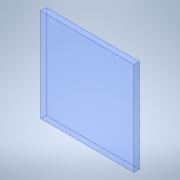
# Autodesk Inventor part: 20_cube_circular_polarizer
Saved by Autodesk Inventor 2022 (Build 260153000, 153)
## iProperties
Created: 2020-10-09
Part Number: 20_cube_circular_polarizer
Material: Generisch
Document SubType Name: Blech
Designer: UC2
Density: 1 g/cm^3
Sheet Metal Rule: Default
Appearance: Vorgabe
Author: UC2
Autodesk Inventor part; units mm, degrees
ref_plane "YZ Plane" through (0, 0, 0) normal (1, 0, 0) x (0, 1, 0)
ref_plane "XZ Plane" through (0, 0, 0) normal (0, 1, 0) x (-1, 0, 0)
ref_plane "XY Plane" through (0, 0, 0) normal (0, 0, 1) x (1, 0, 0)
sketch "Skizze1" plane through (0, 0, 0) normal (0, 0, 1) x (1, 0, 0)
  line L0 (0, 24) -> (0, -24) construction
  line L1 (-17, -17) -> (17, -17)
  line L2 (17, -17) -> (17, 17)
  line L3 (17, 17) -> (-17, 17)
  line L4 (-17, 17) -> (-17, -17)
  line L5 (-17, -17) -> (17, 17) construction
  line L6 (17, -17) -> (-17, 17) construction
  point P0 (0, 0)
  point P1 (0, 0)
  point P2 (0, 0)
  dimension "d4" = 34
  dimension "d5" = 34
  constraints: 16 end point, 4 midpoint, 2 parallel, 1 coincident, 1 horizontal, 1 perpendicular, 1 vertical
  measures "d4" distance of L1.end L2.end
  measures "d5" distance of L2.end L3.end
extrude "Extrusion1" add sketch "Skizze1" along normal blind 2
equation "\"d5\" = d4"
equation "\"Biegeradius\" = Stärke"
equation "\"BreiteBiegungsfreistellung\" = Stärke"
equation "\"TiefeBiegungsfreistellung\" = 0.5 * Stärke"
equation "\"GrößeEckenfreistellung\" = 4 * Stärke"
equation "\"MinimalRest\" = 2 * Stärke"
equation "\"Übergangsradius\" = Biegeradius"
equation "\"JacobiRadiusGröße\" = Biegeradius"
equation "\"Abstandsgröße\" = Stärke"
equation "\"Stärke\" = 3.048"
